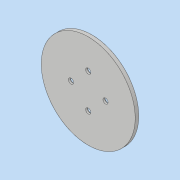
# Autodesk Inventor part: SmallSpoolEndAft
Saved by Autodesk Inventor 2017 (Build 210142000, 142)
## iProperties
Created: 2018-04-03
Part Number: SmallSpoolEndAft
Material: Generic
Document SubType Name: Modeling
Designer: Derek Wider
Density: 1 g/cm^3
Appearance: Default
Author: Derek Wider
Autodesk Inventor part; units mm, degrees
ref_plane "YZ Plane" through (0, 0, 0) normal (1, 0, 0) x (0, 1, 0)
ref_plane "XZ Plane" through (0, 0, 0) normal (0, 1, 0) x (-1, 0, 0)
ref_plane "XY Plane" through (0, 0, 0) normal (0, 0, 1) x (1, 0, 0)
sketch "Sketch1" plane through (0, 0, 0) normal (0, 0, 1) x (1, 0, 0)
  circle A0 centre (0, 0) radius 33.655
  dimension "d0" = 67.31
  constraints: 1 centre point, 1 coincident
  measures "d0" diameter of A0
extrude "Extrusion1" add sketch "Sketch1" along normal blind 2.54
sketch "Sketch2" plane through (0, 0, 0) normal (0, 0, -1) x (-1, 0, 0)
  circle A0 centre (0, 12.3825) radius 1.8415
  point P0 (0, 0)
  dimension "d3" = 3.683
  dimension "d4" = 12.3825
  constraints: 1 centre point
  measures "d3" diameter of A0
  measures "d4" distance of point (0, 0) A0.centre
extrude "Extrusion2" cut sketch "Sketch2" against normal through all
chamfer "Chamfer1" distance 1.27 angle 45 1 edges at (1.8415, 12.3825, 0)
pattern_circular "Circular Pattern1" count 4 over 360 about axis through (0, 0, 0) along (0, 0, 1) of "Extrusion2", "Chamfer1"
body "Solid1"
